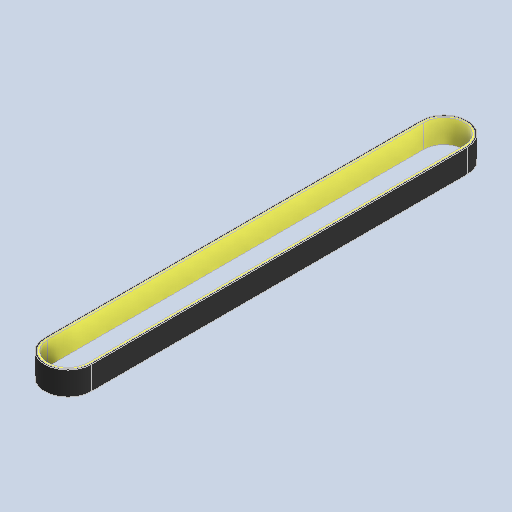
# Autodesk Inventor part: belt1
Saved by Autodesk Inventor 2022 (Build 260153000, 153)
## iProperties
Created: 2022-06-14
Part Number: belt1
Material: ゴム
Document SubType Name: Modeling
Designer: yuto6
Density: 0.93 g/cm^3
Appearance: ゴム - 黒
Author: yuto6
Autodesk Inventor part; units mm, degrees
ref_plane "YZ Plane" through (0, 0, 0) normal (1, 0, 0) x (0, 1, 0)
ref_plane "XZ Plane" through (0, 0, 0) normal (0, 1, 0) x (-1, 0, 0)
ref_plane "XY Plane" through (0, 0, 0) normal (0, 0, 1) x (1, 0, 0)
sketch "スケッチ1" plane through (0, 0, 0) normal (0, 1, 0) x (-1, 0, 0)
  arc A0 (-9.5493, 0) -> (9.5493, 0) centre (0, 0) ccw construction
  arc A1 (9.5493, 160) -> (-9.5493, 160) centre (0, 160) ccw construction
  line L0 (9.5493, 160) -> (9.5493, 0) construction
  line L1 (-9.5493, 160) -> (-9.5493, 0) construction
  line L2 (9.2953, 0) -> (9.2953, 160)
  arc A2 (9.2953, 160) -> (-9.2953, 160) centre (0, 160) ccw
  line L3 (-9.2953, 160) -> (-9.2953, 0)
  arc A3 (-9.2953, 0) -> (9.2953, 0) centre (0, 0) ccw
  line L4 (9.9253, 0) -> (9.9253, 160)
  arc A4 (9.9253, 160) -> (-9.9253, 160) centre (0, 160) ccw
  line L5 (-9.9253, 160) -> (-9.9253, 0)
  arc A5 (-9.9253, 0) -> (9.9253, 0) centre (0, 0) ccw
  dimension "d0" = 19.0986
  dimension "d1" = 19.0986
  dimension "d2" = 160
  dimension "d3" = 0.254
  dimension "d4" = 0.63
  constraints: 12 end point, 12 point on circle, 6 centre point, 4 tangent, 1 coincident, 1 vertical alignment, 6 other
  measures "d0" diameter of A0
  measures "d1" diameter of A1
  measures "d2" distance of A1.centre point (0, 0)
  measures "d3" distance between parallel lines of L2 L0
  measures "d4" distance between parallel lines of L2 L4
extrude "押し出し1" add sketch "スケッチ1" along normal blind 10
sketch "スケッチ2" plane through (0, 0, 0) normal (0, -1, 0) x (1, 0, 0)
  line L0 (9.2953, 0) -> (9.2953, 160) projected
  arc A0 (9.2953, 160) -> (-9.2953, 160) centre (0, 160) ccw projected
  line L1 (9.2953, 0) -> (9.2953, 160)
  line L2 (-9.2953, 160) -> (-9.2953, 0) projected
  line L3 (-9.2953, 160) -> (-9.2953, 0)
  arc A1 (-9.2953, 0) -> (9.2953, 0) centre (0, 0) ccw projected
  arc A2 (-9.2953, 0) -> (9.2953, 0) centre (0, 0) ccw
  arc A3 (9.2953, 160) -> (-9.2953, 160) centre (0, 160) ccw
  line L4 (8.5453, 160) -> (8.5453, 0)
  arc A4 (-8.5453, 0) -> (8.5453, 0) centre (0, 0) ccw
  line L5 (-8.5453, 0) -> (-8.5453, 160)
  arc A5 (8.5453, 160) -> (-8.5453, 160) centre (0, 160) ccw
  dimension "d7" = 0.75
  constraints: 8 end point, 8 point on circle, 4 centre point, 2 coincident, 1 collinear, 1 concentric, 1 tangent, 1 vertical, 3 other
  measures "d7" distance between parallel lines of L0 L4
extrude "押し出し2" add sketch "スケッチ2" against normal blind 10 separate body
equation "\"d1\" = d0"
